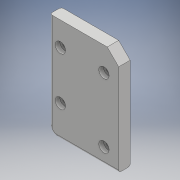
# Autodesk Inventor part: bearing bracket for bolt screw
Saved by Autodesk Inventor 2018 (Build 220112000, 112)
## iProperties
Created: 2018-04-10
Part Number: bearing bracket for bolt screw
Material: Generic
Document SubType Name: Modeling
Designer: m234676
Density: 1 g/cm^3
Appearance: Default
Author: m234676
Autodesk Inventor part; units mm, degrees
ref_plane "YZ Plane" through (0, 0, 0) normal (1, 0, 0) x (0, 1, 0)
ref_plane "XZ Plane" through (0, 0, 0) normal (0, 1, 0) x (-1, 0, 0)
ref_plane "XY Plane" through (0, 0, 0) normal (0, 0, 1) x (1, 0, 0)
sketch "Sketch2" plane through (0, 0, 0) normal (0, 1, 0) x (-1, 0, 0)
  line L0 (0, 0) -> (60, 0)
  line L1 (60, 0) -> (60, -90)
  line L2 (60, -90) -> (0, -90)
  line L3 (0, -90) -> (0, 0)
  dimension "d5" = 60
  dimension "d6" = 90
  constraints: 8 end point, 2 parallel, 1 horizontal, 1 perpendicular
  measures "d5" distance of L1.end L2.end
  measures "d6" distance of L0.end L1.end
extrude "Extrusion1" add sketch "Sketch2" along normal mid plane 10
sketch "Sketch3" plane through (0, 5, 0) normal (0, 1, 0) x (1, 0, 0)
  line L0 (-60, 0) -> (0, 0) construction
  line L1 (0, 0) -> (-31.8198, 31.8198) construction
  line L2 (0, 0) -> (45, 0) construction
  circle A0 centre (-31.8198, 31.8198) radius 12
  dimension "d9" = 45
  dimension "d10" = 135
  dimension "d11" = 24
  constraints: 4 end point, 1 centre point, 1 coincident, 1 equal length, 1 horizontal
  measures "d9" distance of L0.end L1.end
  measures "d10" angle of L2 L1
  measures "d11" diameter of A0
extrude "Extrusion2" cut sketch "Sketch3" against normal blind 2
chamfer "Chamfer1" distance 10 angle 45 1 edges at (0, 0, 0)
fillet "Fillet1" radius 6 1 edges at (-60, 0, -90)
fillet "Fillet1" radius 2 4 edges at (-30, 5, -90) (-30, -5, -90) (-60, -5, -45) (-60, 5, -45)
sketch "Sketch4" plane through (0, 5, 0) normal (0, 1, 0) x (1, 0, 0)
  circle A0 centre (-31.8198, 31.8198) radius 12 projected
  line L0 (-31.8198, 31.8198) -> (-12.8198, 31.8198) construction
  line L1 (-12.8198, 31.8198) -> (-12.8198, 20.8198) construction
  circle A1 centre (-12.8198, 20.8198) radius 2
  line L2 (-31.8198, 31.8198) -> (-31.8198, 62.8198) construction
  line L3 (-31.8198, 31.8198) -> (-31.8198, 76.8198) construction
  circle A2 centre (-50.8198, 20.8198) radius 2
  line L4 (-31.8198, 76.8198) -> (-12.8198, 76.8198) construction
  line L5 (-31.8198, 62.8198) -> (-50.8198, 62.8198) construction
  circle A3 centre (-12.8198, 76.8198) radius 2
  circle A4 centre (-50.8198, 62.8198) radius 2
  point P0 (0, 0)
  dimension "d19" = 19
  dimension "d20" = 11
  dimension "d21" = 4
  dimension "d22" = 31
  dimension "d30" = 19
  dimension "d32" = 19
  dimension "d33" = 45
  dimension "d34" = 4
  dimension "d35" = 4
  constraints: 12 end point, 4 centre point, 3 coincident, 2 horizontal, 2 perpendicular, 1 parallel, 1 symmetric about line, 1 vertical, 1 other
  measures "d19" distance of L0.start L0.end
  measures "d20" distance of L0.end L1.end
  measures "d21" diameter of A1
  measures "d22" distance of L0.start L2.end
  measures "d30" distance of L3.end L4.end
  measures "d32" distance of L2.end L5.end
  measures "d33" distance between parallel lines of L4 L0
  measures "d34" diameter of A3
  measures "d35" diameter of A4
extrude "Extrusion4" cut sketch "Sketch4" against normal up to surface (10 mm away) contours A1 | A2 | A3 | A4
sketch "Sketch6" plane through (0, -5, 0) normal (0, -1, 0) x (1, 0, 0)
  circle A0 centre (-50.8198, -20.8198) radius 2 projected
  circle A1 centre (-12.8198, -20.8198) radius 2 projected
  circle A2 centre (-50.8198, -62.8198) radius 2 projected
  circle A3 centre (-12.8198, -76.8198) radius 2 projected
  circle A4 centre (-50.8198, -20.8198) radius 2 projected
  circle A5 centre (-50.8198, -20.8198) radius 4.5
  circle A6 centre (-12.8198, -20.8198) radius 2 projected
  circle A7 centre (-12.8198, -20.8198) radius 4.5
  circle A8 centre (-50.8198, -62.8198) radius 4.5
  circle A9 centre (-12.8198, -76.8198) radius 2 projected
  circle A10 centre (-12.8198, -76.8198) radius 4.5
  point P0 (0, 0)
  dimension "d45" = 9
  dimension "d46" = 9
  dimension "d47" = 9
  dimension "d48" = 9
  constraints: 4 centre point, 4 coincident
  measures "d45" diameter of A5
  measures "d46" diameter of A7
  measures "d47" diameter of A8
  measures "d48" diameter of A10
extrude "Extrusion6" cut sketch "Sketch6" against normal blind 4
sketch "Sketch7" plane through (0, 5, 0) normal (0, 1, 0) x (1, 0, 0)
  circle A0 centre (-12.8198, 20.8198) radius 2 projected
  circle A1 centre (-50.8198, 20.8198) radius 2 projected
  circle A2 centre (-50.8198, 62.8198) radius 2 projected
  circle A3 centre (-12.8198, 76.8198) radius 2 projected
  circle A4 centre (-12.8198, 20.8198) radius 2 projected
  circle A5 centre (-12.8198, 20.8198) radius 5
  circle A6 centre (-50.8198, 20.8198) radius 5
  circle A7 centre (-12.8198, 76.8198) radius 5
  circle A8 centre (-50.8198, 62.8198) radius 5
  point P0 (0, 0)
  dimension "d51" = 10
  dimension "d52" = 10
  dimension "d53" = 10
  dimension "d54" = 10
  constraints: 4 centre point, 4 coincident
  measures "d51" diameter of A5
  measures "d52" diameter of A6
  measures "d53" diameter of A7
  measures "d54" diameter of A8
extrude "Extrusion7" cut sketch "Sketch7" against normal blind 1
thread "Thread1" size "M4x0.7" class "6H" standard "ANSI Metric M Profile" full length
thread "Thread2" size "M4x0.7" class "6H" standard "ANSI Metric M Profile" full length
thread "Thread3" size "M4x0.7" class "6H" standard "ANSI Metric M Profile" full length
thread "Thread4" size "M4x0.7" class "6H" standard "ANSI Metric M Profile" full length
body "Solid1"
